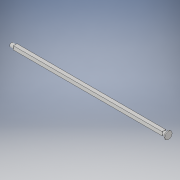
# Autodesk Inventor part: MotorMntPart
Saved by Autodesk Inventor 2017 (Build 210142000, 142)
## iProperties
Created: 2017-01-26
Part Number: MotorMntPart
Material: Generic
Document SubType Name: Modeling
Designer: David Kopala
Density: 1 g/cm^3
Appearance: Default
Author: David Kopala
Autodesk Inventor part; units mm, degrees
ref_plane "YZ Plane" through (0, 0, 0) normal (1, 0, 0) x (0, 1, 0)
ref_plane "XZ Plane" through (0, 0, 0) normal (0, 1, 0) x (-1, 0, 0)
ref_plane "XY Plane" through (0, 0, 0) normal (0, 0, 1) x (1, 0, 0)
sketch "Sketch1" plane through (0, 0, 0) normal (0, 1, 0) x (-1, 0, 0)
  line L0 (0, 0) -> (260.0718, 0)
  line L1 (260.0718, 0) -> (260.0718, -6.35)
  line L2 (260.0718, -6.35) -> (0, -6.35)
  line L3 (0, -6.35) -> (0, 0)
  dimension "d0" = 260.0718
  dimension "d1" = 6.35
  constraints: 8 end point, 2 parallel, 1 horizontal, 1 perpendicular
  measures "d0" distance of L1.end L2.end
  measures "d1" distance of L2.end L0.start
extrude "Extrusion1" add sketch "Sketch1" along normal blind 6.35
sketch "Sketch2" plane through (-260.0718, 0, -6.35) normal (-1, 0, 0) x (0, 0, 1)
  line L0 (6.35, 6.35) -> (0, 6.35) projected
  line L1 (6.35, 0) -> (6.35, 6.35) projected
  circle A0 centre (3.175, 3.175) radius 3.175
  dimension "d4" = 3.175
  dimension "d5" = 3.175
  dimension "d6" = 6.35
  constraints: 1 centre point, 1 coincident
  measures "d4" distance from line of L0 point (3.175, 3.175)
  measures "d5" distance from line of L1 point (3.175, 3.175)
  measures "d6" diameter of A0
extrude "Extrusion2" add sketch "Sketch2" along normal blind 6.35 contours A0
sketch "Sketch3" plane through (0, 0, 0) normal (1, 0, 0) x (0, 0, -1)
  line L0 (0, 6.35) -> (6.35, 6.35) projected
  line L1 (6.35, 0) -> (6.35, 6.35) projected
  circle A0 centre (3.175, 3.175) radius 3.175
  point P0 (0, 0)
  dimension "d9" = 3.175
  dimension "d10" = 3.175
  dimension "d11" = 6.35
  constraints: 1 centre point, 1 coincident
  measures "d9" distance from line of L0 point (3.175, 3.175)
  measures "d10" distance from line of L1 point (3.175, 3.175)
  measures "d11" diameter of A0
extrude "Extrusion3" add sketch "Sketch3" along normal blind 6.35 contours A0
sketch "Sketch4" plane through (6.35, 3.175, -3.175) normal (1, 0, 0) x (0, 0, -1)
  circle A0 centre (0, 0) radius 6.35
  point P0 (-3.175, -3.175)
  dimension "d14" = 12.7
  constraints: 1 centre point
  measures "d14" diameter of A0
extrude "Extrusion4" add sketch "Sketch4" along normal blind 1.5875
equation "\"d0\" = -6 * SpWall + IBDia"
equation "\"d1\" = AxelDia"
equation "\"d2\" = AxelDia"
equation "\"d4\" = 0.5 * AxelDia"
equation "\"d5\" = 0.5 * AxelDia"
equation "\"d6\" = AxelDia"
equation "\"d7\" = 2 * SpWall"
equation "\"d9\" = 0.5 * AxelDia"
equation "\"d10\" = 0.5 * AxelDia"
equation "\"d11\" = AxelDia"
equation "\"d12\" = 2 * SpWall"
equation "\"d15\" = Wall"
equation "\"SpWall\" = 3.175"
equation "\"IBDia\" = 279.121792"
equation "\"AxelDia\" = 6.35"
equation "\"Wall\" = 1.5875"
body "Solid1"
